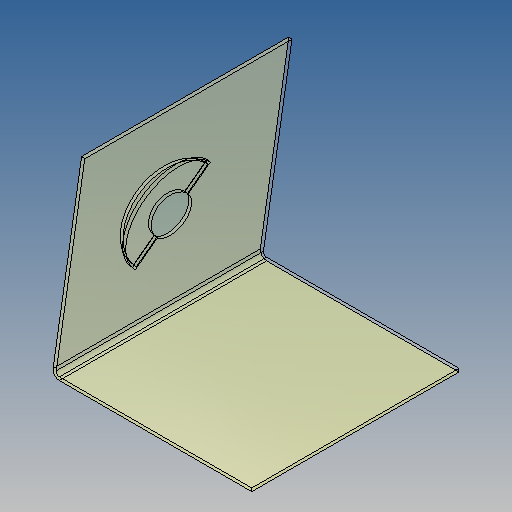
# Autodesk Inventor part: tapa
Saved by Autodesk Inventor 2017 (Build 210142000, 142)
## iProperties
Created: 2017-08-05
Part Number: tapa
Material: Polycarbonate, Clear
Document SubType Name: Sheet Metal
Designer: leo
Density: 1.2 g/cm^3
Appearance: Polycarbonate - Clear
Sheet Metal Rule: Default
Author: leo
Autodesk Inventor part; units mm, degrees
ref_plane "YZ Plane" through (0, 0, 0) normal (1, 0, 0) x (0, 1, 0)
ref_plane "XZ Plane" through (0, 0, 0) normal (0, 1, 0) x (-1, 0, 0)
ref_plane "XY Plane" through (0, 0, 0) normal (0, 0, 1) x (1, 0, 0)
sketch "Sketch1" plane through (0, 0, 0) normal (0, 0, 1) x (1, 0, 0)
  line L0 (-31.4741, 49) -> (-44.9693, -44.5718)
  arc A0 (-44.9693, -44.5718) -> (-42, -48) centre (-42, -45) ccw
  line L1 (-42, -48) -> (49, -48)
  line L2 (-45, -39.9809) -> (-45, -2.5) construction
  circle A1 centre (-35.5147, 42) radius 2 construction
  circle A2 centre (-35.5147, 42) radius 3 construction
  point P0 (0, 0)
  dimension "d0" = 49
  dimension "d1" = 49
  dimension "d2" = 48
  dimension "d3" = 45
  dimension "d4" = 6
  dimension "d5" = 3
  constraints: 6 end point, 4 tangent, 2 centre point, 2 point on circle, 1 coincident, 1 horizontal, 1 vertical
  measures "d0" vertical distance of L0.start point (0, 0)
  measures "d1" horizontal distance of L1.end point (0, 0)
  measures "d2" vertical distance of L1.end point (0, 0)
  measures "d3" distance from line of point (0, 0) L2
  measures "d4" diameter of A2
  measures "d5" radius of A0
surface extrude "ExtrusionSrf1" sketch "Sketch1" along normal mid plane 98 shown yes curves L0 A0 L1
thicken "Thicken1" operation new thickness 1.5 both sides no extend neighbours no toward (0.9897594, -0.1427456, 0) faces at (-35.9725, 17.8094, 16.3333) (-44.9498, -45.5467, 16.3333) (-11.6667, -48, -16.3333)
sketch "Sketch2" plane through (-44.9693, -44.5718, -49) normal (-0.9897594, 0.1427456, 0) x (0, 0, 1)
  line L0 (34.1508, 57.3837) -> (63.8492, 27.6852)
  arc A0 (64.5563, 26.9781) -> (33.4437, 58.0908) centre (49, 42.5345) ccw
  arc A1 (63.8492, 27.6852) -> (34.1508, 57.3837) centre (49, 42.5345) ccw
  arc A2 (33.4437, 58.0908) -> (34.1508, 57.3837) centre (33.7972, 57.7373) ccw
  arc A3 (63.8492, 27.6852) -> (64.5563, 26.9781) centre (64.2028, 27.3317) ccw
  line L1 (49, 74.7006) -> (49, 10.3683) construction
  point P0 (49, 50.5345)
  dimension "d9" = 1
  dimension "d10" = 315
  dimension "d11" = 21
  dimension "d12" = 8
  constraints: 8 point on circle, 4 centre point, 4 end point, 4 tangent, 2 midpoint, 1 point on line, 1 vertical
  measures "d9" radial gap between concentric circles of A0 A1
  measures "d11" radius of A1
  measures "d12" distance of A0.centre point (49, 50.534)
extrude "Extrusion1" cut sketch "Sketch2" against normal up to next contours A2 A0 A3 A1
fold "Fold1" angle 10 bend radius 1.5 thickness 1.5 k factor 0.44 line from (-36.778, 12.2243, -14.8492) to (-41.0173, -17.17, 14.8492) line at bend centre moving side (0.1009364, 0.6998656, 0.7071068) folds toward (-0.9897594, 0.1427456, 0)
sketch "Sketch3" plane through (-38.8993, -2.5538, -0.0804) normal (-0.9922502, 0.0190466, -0.1227878) x (-0.1009364, -0.6998656, 0.7071068)
  arc A0 (20.9992, 0.1885) -> (-20.9992, 0.1885) centre (0, 0) ccw construction
  circle A1 centre (0, 0) radius 9
  point P0 (-5.6569, -0.9395)
  dimension "d21" = 18
  constraints: 1 centre point, 1 coincident
  measures "d21" diameter of A1
extrude "Extrusion2" cut sketch "Sketch3" along normal through all both and the other way through all
equation "\"d1\" = d0"
equation "\"d15\" = BendReliefWidth"
equation "\"d16\" = BendReliefDepth"
equation "\"d17\" = MinimumRemnant"
equation "\"d18\" = BendRadius"
equation "\"d20\" = BendRadius"
equation "\"BendRadius\" = Thickness"
equation "\"BendReliefWidth\" = Thickness"
equation "\"BendReliefDepth\" = 0.5 * Thickness"
equation "\"CornerReliefSize\" = 4 * Thickness"
equation "\"MinimumRemnant\" = 2 * Thickness"
equation "\"TransitionRadius\" = BendRadius"
equation "\"JacobiRadiusSize\" = Thickness"
equation "\"GapSize\" = Thickness"
equation "\"Thickness\" = 1.5"
body "Solid1"
body "Srf1"
